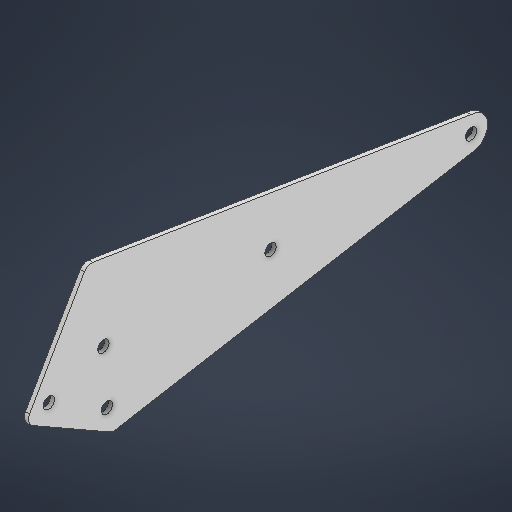
# Autodesk Inventor part: preroller
Saved by Autodesk Inventor 2025.2 (Build 292293000, 293)
## iProperties
Created: 2025-03-30
Part Number: preroller
Material: Generic
Document SubType Name: Modeling
Designer: roejo
Density: 1 g/cm^3
Appearance: Default
Author: roejo
Autodesk Inventor part; units mm, degrees
ref_plane "YZ Plane" through (0, 0, 0) normal (1, 0, 0) x (0, 1, 0)
ref_plane "XZ Plane" through (0, 0, 0) normal (0, 1, 0) x (-1, 0, 0)
ref_plane "XY Plane" through (0, 0, 0) normal (0, 0, 1) x (1, 0, 0)
sketch "Sketch1" plane through (0, 0, 0) normal (1, 0, 0) x (0, 1, 0)
  circle A0 centre (1.2483, -80.7841) radius 2.1844
  circle A1 centre (1.2483, -80.7841) radius 6.35
  line L0 (7.5983, -80.7841) -> (30.8366, 62.9)
  line L1 (29.2789, 66.1628) -> (-7.1078, 86.9787)
  line L2 (-28.5868, 54.3573) -> (-5.1017, -80.7841)
  circle A2 centre (-7.0352, 79.6215) radius 2.1844
  circle A3 centre (-19.6479, 57.5743) radius 2.1844
  line L3 (-11.4403, 85.7994) -> (-28.2146, 56.4775)
  arc A4 (-7.1078, 86.9787) -> (-11.4403, 85.7994) centre (-8.6844, 84.2228) ccw
  arc A5 (30.8366, 62.9) -> (29.2789, 66.1628) centre (27.7024, 63.4069) ccw
  arc A6 (-28.2146, 56.4775) -> (-28.5868, 54.3573) centre (-25.4587, 54.9009) ccw
  circle A7 centre (1.2483, 58.9159) radius 2.1844
  circle A8 centre (1.2483, -4.5841) radius 2.1844
  point P0 (0, 0)
  point P1 (-9.8637, 88.5553)
  point P2 (-28.7827, 55.4844)
  dimension "d0" = 12.7
  dimension "d1" = 38.1
  dimension "d2" = 4.3688
  dimension "d3" = 4.3688
  dimension "d4" = 3.175
  dimension "d5" = 3.175
  constraints: 9 centre point, 8 end point, 8 point on circle, 6 tangent, 4 point on line, 1 coincident, 1 equal radius
  measures "d0" diameter of A1
  measures "d1" distance of point (-9.864, 88.555) point (-28.783, 55.484)
  measures "d2" diameter of A2
  measures "d3" diameter of A3
  measures "d4" radius of A4
  measures "d5" radius of A5
extrude "Extrusion1" add sketch "Sketch1" along normal blind 1.5875
body "Solid1"
